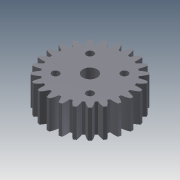
# Autodesk Inventor part: Spur Gear1
Saved by Autodesk Inventor 2015 (Build 190159000, 159)
## iProperties
Created: 2014-08-31
Part Number: Spur Gear1
Material: Steel
Document SubType Name: Modeling
Designer: shohei
Categories: <?xml version="1.0" encoding="UTF-16"?> <MemberInstance><Categories><FamilyTemplate><FamilyTemplateParameter ValueType="xs:double" Id="1" ObjectReferenceKey="da_z" ObjectType="kUserParameterObject"/><FamilyTemplateParameter ValueType="xs:double" Id="2" ObjectReferenceKey="da_b" ObjectType="kUserParameterObject"/><FamilyTemplateParameter ValueType="xs:double" Id="3" ObjectReferenceKey="da_beta" ObjectType="kUserParameterObject"/><FamilyTemplateParameter ValueType="xs:double" Id="4" ObjectReferenceKey="da_da" ObjectType="kUserParameterObject"/><FamilyTemplateParameter ValueType="xs:double" Id="5" ObjectReferenceKey="da_aw" ObjectType="kUserParameterObject"/><FamilyTemplateParameter ValueType="xs:string" Id="6" ObjectReferenceKey="EAIAABAAAACIAQAAAAAAAIAAAAAAAAAA" ObjectType="83910656" SubObjectId="SurfaceGeometry"/></FamilyTemplate><ParamToTemplateMap><ParamToTemplate CategoryParameter="//CategoryParameter[@InternalName='046C89C9-8512-4d59-83FE-43B91F4F132A']" TemplateParameter="1"/><ParamToTemplate CategoryParameter="//CategoryParameter[@InternalName='2552DF32-E462-4b46-AEBF-C6C7768E72AC']" TemplateParameter="2"/><ParamToTemplate CategoryParameter="//CategoryParameter[@InternalName='C9EE641D-15FC-4fae-A226-E94C4372FDD7']" TemplateParameter="3"/><ParamToTemplate><ParamToTemplate CategoryParameter="//CategoryParameter[@InternalName='00B6519A-459B-49c7-AD84-2E56D39A5744']" ConstantValue="0.000000"/></ParamToTemplate><ParamToTemplate><ParamToTemplate CategoryParameter="//CategoryParameter[@InternalName='04B31F0E-C7A6-4894-AA32-9629BEFACF47']" ConstantValue="1.000000"/></ParamToTemplate><ParamToTemplate><ParamToTemplate CategoryParameter="//CategoryParameter[@InternalName='43CBEC2E-7847-49e7-A936-2F7889FCB2D9']" ConstantValue="0.250000"/></ParamToTemplate><ParamToTemplate><ParamToTemplate CategoryParameter="//CategoryParameter[@InternalName='B1EFC894-105D-4ebd-86BF-FA20ED196853']" ConstantValue="0.350000"/></ParamToTemplate><ParamToTemplate><ParamToTemplate CategoryParameter="//CategoryParameter[@InternalName='51175063-3D10-4879-93E8-6246FE8B403D']" ConstantValue="2060000000.000000"/></ParamToTemplate><ParamToTemplate><ParamToTemplate CategoryParameter="//CategoryParameter[@InternalName='A3A52E27-4454-46a9-B0BD-C932399B70AF']" ConstantValue="0.300000"/></ParamToTemplate><ParamToTemplate><ParamToTemplate CategoryParameter="//CategoryParameter[@InternalName='91B76062-C214-41d9-B1B9-14D2AB99603D']" ConstantValue="0.225000"/></ParamToTemplate><ParamToTemplate><ParamToTemplate CategoryParameter="//CategoryParameter[@InternalName='374E806E-8B8A-4dda-A9AA-1039D6500AD2']" ConstantValue="4.444444"/></ParamToTemplate><ParamToTemplate><ParamToTemplate CategoryParameter="//CategoryParameter[@InternalName='2D373A89-B862-43d6-8D0B-0CBF12AB9F6C']" ConstantValue="0.349066"/></ParamToTemplate><ParamToTemplate CategoryParameter="//CategoryParameter[@InternalName='37777632-D6A2-4fac-9D53-DB8ACD95C989']" TemplateParameter="4"/><ParamToTemplate CategoryParameter="//CategoryParameter[@InternalName='FD1017F1-B727-4f7e-9707-0F86F1FF9423']" TemplateParameter="5"/><ParamToTemplate><ParamToTemplate CategoryParameter="//CategoryParameter[@InternalName='9E1B4470-B2D3-4ff1-B813-535BB4CDF51A']" ConstantValue="3520000.000000"/></ParamToTemplate><ParamToTemplate><ParamToTemplate CategoryParameter="//CategoryParameter[@InternalName='F8452263-BFF6-458c-9FB1-07C4B99E95CD']" ConstantValue="11400000.000000"/></ParamToTemplate><ParamToTemplate><ParamToTemplate CategoryParameter="//CategoryParameter[@InternalName='3E3BB259-FD49-497f-8171-6EBC954A3479']" ConstantValue="2.000000"/></ParamToTemplate><ParamToTemplate CategoryParameter="//CategoryParameter[@InternalName='27C3BAF2-7550-4e4b-AE2C-0DB134B7D9B7']" TemplateParameter="6"/></ParamToTemplateMap><Category DisplayName="Gear" InternalName="DC85795E-93AB-48d5-8EEE-5A27447B64BD" Mnemonic="Gear"><CategoryParameter DisplayName="z" InternalName="046C89C9-8512-4d59-83FE-43B91F4F132A" Mnemonic="z"/><CategoryParameter DisplayName="b" InternalName="2552DF32-E462-4b46-AEBF-C6C7768E72AC" Mnemonic="b"/><CategoryParameter DisplayName="||b|" InternalName="C9EE641D-15FC-4fae-A226-E94C4372FDD7" Mnemonic="beta"/><CategoryParameter DisplayName="x" InternalName="00B6519A-459B-49c7-AD84-2E56D39A5744" Mnemonic="x"/><CategoryParameter DisplayName="a*" InternalName="04B31F0E-C7A6-4894-AA32-9629BEFACF47" Mnemonic="a"/><CategoryParameter DisplayName="c*" InternalName="43CBEC2E-7847-49e7-A936-2F7889FCB2D9" Mnemonic="c"/><CategoryParameter DisplayName="r|.f|*" InternalName="B1EFC894-105D-4ebd-86BF-FA20ED196853" Mnemonic="rf"/><CategoryParameter DisplayName="E" InternalName="51175063-3D10-4879-93E8-6246FE8B403D" Mnemonic="E"/><CategoryParameter DisplayName="||m|" InternalName="A3A52E27-4454-46a9-B0BD-C932399B70AF" Mnemonic="mi"/><Category DisplayName="SpurGear" InternalName="26C5A22E-A91E-4dfd-A3B3-23CCAFAE1764" Mnemonic="SpurGear"><CategoryParameter DisplayName="m" InternalName="91B76062-C214-41d9-B1B9-14D2AB99603D" Mnemonic="m"/><CategoryParameter DisplayName="P" InternalName="374E806E-8B8A-4dda-A9AA-1039D6500AD2" Mnemonic="PP"/><CategoryParameter DisplayName="||a|" InternalName="2D373A89-B862-43d6-8D0B-0CBF12AB9F6C" Mnemonic="alpha"/><CategoryParameter DisplayName="d|.a|" InternalName="37777632-D6A2-4fac-9D53-DB8ACD95C989" Mnemonic="da"/><CategoryParameter DisplayName="a|.w|" InternalName="FD1017F1-B727-4f7e-9707-0F86F1FF9423" Mnemonic="aw"/><CategoryParameter DisplayName="||s||.Flim|" InternalName="9E1B4470-B2D3-4ff1-B813-535BB4CDF51A" Mnemonic="sFlim"/><CategoryParameter DisplayName="||s||.Hlim|" InternalName="F8452263-BFF6-458c-9FB1-07C4B99E95CD" Mnemonic="sHlim"/><CategoryParameter DisplayName="type" InternalName="3E3BB259-FD49-497f-8171-6EBC954A3479" Mnemonic="type"/><CategoryParameter DisplayName="PitchDiameter" InternalName="27C3BAF2-7550-4e4b-AE2C-0DB134B7D9B7" Mnemonic="IDS_PITCHDIAM"/></Category></Category></Categories></MemberInstance>
Density: 1 g/cm^3
Appearance: Steel
CustomPartVersion: 1
Author: shohei
Autodesk Inventor part; units mm, degrees
sketch "Block1" plane through (0, 0, 0) normal (0, 0, 1) x (1, 0, 0)
  arc A0 (1.1045, 29.446) -> (-1.1045, 29.446) centre (0, 0) ccw
  arc A1 (2.5646, 24.2724) -> (1.1045, 29.446) centre (-17.8247, 21.311) ccw
  arc A2 (3.805, 24.1091) -> (2.5646, 24.2724) centre (0, 0) ccw
  arc A3 (6.5543, 28.7285) -> (3.805, 24.1091) centre (22.733, 15.9715) ccw
  arc A4 (8.6881, 28.1567) -> (6.5543, 28.7285) centre (0, 0) ccw
  arc A5 (8.7594, 22.7816) -> (8.6881, 28.1567) centre (-11.7016, 25.1982) ccw
  arc A6 (9.9152, 22.3028) -> (8.7594, 22.7816) centre (0, 0) ccw
  arc A7 (13.7664, 26.0532) -> (9.9152, 22.3028) centre (26.0921, 9.5435) ccw
  arc A8 (15.6795, 24.9487) -> (13.7664, 26.0532) centre (0, 0) ccw
  arc A9 (14.3572, 19.7382) -> (15.6795, 24.9487) centre (-4.7811, 27.3682) ccw
  arc A10 (15.3497, 18.9766) -> (14.3572, 19.7382) centre (0, 0) ccw
  arc A11 (20.0404, 21.6024) -> (15.3497, 18.9766) centre (27.6731, 2.4652) ccw
  arc A12 (21.6024, 20.0404) -> (20.0404, 21.6024) centre (0, 0) ccw
  arc A13 (18.9766, 15.3497) -> (21.6024, 20.0404) centre (2.4652, 27.6731) ccw
  arc A14 (19.7382, 14.3572) -> (18.9766, 15.3497) centre (0, 0) ccw
  arc A15 (24.9487, 15.6795) -> (19.7382, 14.3572) centre (27.3682, -4.7811) ccw
  arc A16 (26.0532, 13.7664) -> (24.9487, 15.6795) centre (0, 0) ccw
  arc A17 (22.3028, 9.9152) -> (26.0532, 13.7664) centre (9.5435, 26.0921) ccw
  arc A18 (22.7816, 8.7594) -> (22.3028, 9.9152) centre (0, 0) ccw
  arc A19 (28.1567, 8.6881) -> (22.7816, 8.7594) centre (25.1982, -11.7016) ccw
  arc A20 (28.7285, 6.5543) -> (28.1567, 8.6881) centre (0, 0) ccw
  arc A21 (24.1091, 3.805) -> (28.7285, 6.5543) centre (15.9715, 22.733) ccw
  arc A22 (24.2724, 2.5646) -> (24.1091, 3.805) centre (0, 0) ccw
  arc A23 (29.446, 1.1045) -> (24.2724, 2.5646) centre (21.311, -17.8247) ccw
  arc A24 (29.446, -1.1045) -> (29.446, 1.1045) centre (0, 0) ccw
  arc A25 (24.2724, -2.5646) -> (29.446, -1.1045) centre (21.311, 17.8247) ccw
  arc A26 (24.1091, -3.805) -> (24.2724, -2.5646) centre (0, 0) ccw
  arc A27 (28.7285, -6.5543) -> (24.1091, -3.805) centre (15.9715, -22.733) ccw
  arc A28 (28.1567, -8.6881) -> (28.7285, -6.5543) centre (0, 0) ccw
  arc A29 (22.7816, -8.7594) -> (28.1567, -8.6881) centre (25.1982, 11.7016) ccw
  arc A30 (22.3028, -9.9152) -> (22.7816, -8.7594) centre (0, 0) ccw
  arc A31 (26.0532, -13.7664) -> (22.3028, -9.9152) centre (9.5435, -26.0921) ccw
  arc A32 (24.9487, -15.6795) -> (26.0532, -13.7664) centre (0, 0) ccw
  arc A33 (19.7382, -14.3572) -> (24.9487, -15.6795) centre (27.3682, 4.7811) ccw
  arc A34 (18.9766, -15.3497) -> (19.7382, -14.3572) centre (0, 0) ccw
  arc A35 (21.6024, -20.0404) -> (18.9766, -15.3497) centre (2.4652, -27.6731) ccw
  arc A36 (20.0404, -21.6024) -> (21.6024, -20.0404) centre (0, 0) ccw
  arc A37 (15.3497, -18.9766) -> (20.0404, -21.6024) centre (27.6731, -2.4652) ccw
  arc A38 (14.3572, -19.7382) -> (15.3497, -18.9766) centre (0, 0) ccw
  arc A39 (15.6795, -24.9487) -> (14.3572, -19.7382) centre (-4.7811, -27.3682) ccw
  arc A40 (13.7664, -26.0532) -> (15.6795, -24.9487) centre (0, 0) ccw
  arc A41 (9.9152, -22.3028) -> (13.7664, -26.0532) centre (26.0921, -9.5435) ccw
  arc A42 (8.7594, -22.7816) -> (9.9152, -22.3028) centre (0, 0) ccw
  arc A43 (8.6881, -28.1567) -> (8.7594, -22.7816) centre (-11.7016, -25.1982) ccw
  arc A44 (6.5543, -28.7285) -> (8.6881, -28.1567) centre (0, 0) ccw
  arc A45 (3.805, -24.1091) -> (6.5543, -28.7285) centre (22.733, -15.9715) ccw
  arc A46 (2.5646, -24.2724) -> (3.805, -24.1091) centre (0, 0) ccw
  arc A47 (1.1045, -29.446) -> (2.5646, -24.2724) centre (-17.8247, -21.311) ccw
  arc A48 (-1.1045, -29.446) -> (1.1045, -29.446) centre (0, 0) ccw
  arc A49 (-2.5646, -24.2724) -> (-1.1045, -29.446) centre (17.8247, -21.311) ccw
  arc A50 (-3.805, -24.1091) -> (-2.5646, -24.2724) centre (0, 0) ccw
  arc A51 (-6.5543, -28.7285) -> (-3.805, -24.1091) centre (-22.733, -15.9715) ccw
  arc A52 (-8.6881, -28.1567) -> (-6.5543, -28.7285) centre (0, 0) ccw
  arc A53 (-8.7594, -22.7816) -> (-8.6881, -28.1567) centre (11.7016, -25.1982) ccw
  arc A54 (-9.9152, -22.3028) -> (-8.7594, -22.7816) centre (0, 0) ccw
  arc A55 (-13.7664, -26.0532) -> (-9.9152, -22.3028) centre (-26.0921, -9.5435) ccw
  arc A56 (-15.6795, -24.9487) -> (-13.7664, -26.0532) centre (0, 0) ccw
  arc A57 (-14.3572, -19.7382) -> (-15.6795, -24.9487) centre (4.7811, -27.3682) ccw
  arc A58 (-15.3497, -18.9766) -> (-14.3572, -19.7382) centre (0, 0) ccw
  arc A59 (-20.0404, -21.6024) -> (-15.3497, -18.9766) centre (-27.6731, -2.4652) ccw
  arc A60 (-21.6024, -20.0404) -> (-20.0404, -21.6024) centre (0, 0) ccw
  arc A61 (-18.9766, -15.3497) -> (-21.6024, -20.0404) centre (-2.4652, -27.6731) ccw
  arc A62 (-19.7382, -14.3572) -> (-18.9766, -15.3497) centre (0, 0) ccw
  arc A63 (-24.9487, -15.6795) -> (-19.7382, -14.3572) centre (-27.3682, 4.7811) ccw
  arc A64 (-26.0532, -13.7664) -> (-24.9487, -15.6795) centre (0, 0) ccw
  arc A65 (-22.3028, -9.9152) -> (-26.0532, -13.7664) centre (-9.5435, -26.0921) ccw
  arc A66 (-22.7816, -8.7594) -> (-22.3028, -9.9152) centre (0, 0) ccw
  arc A67 (-28.1567, -8.6881) -> (-22.7816, -8.7594) centre (-25.1982, 11.7016) ccw
  arc A68 (-28.7285, -6.5543) -> (-28.1567, -8.6881) centre (0, 0) ccw
  arc A69 (-24.1091, -3.805) -> (-28.7285, -6.5543) centre (-15.9715, -22.733) ccw
  arc A70 (-24.2724, -2.5646) -> (-24.1091, -3.805) centre (0, 0) ccw
  arc A71 (-29.446, -1.1045) -> (-24.2724, -2.5646) centre (-21.311, 17.8247) ccw
  arc A72 (-29.446, 1.1045) -> (-29.446, -1.1045) centre (0, 0) ccw
  arc A73 (-24.2724, 2.5646) -> (-29.446, 1.1045) centre (-21.311, -17.8247) ccw
  arc A74 (-24.1091, 3.805) -> (-24.2724, 2.5646) centre (0, 0) ccw
  arc A75 (-28.7285, 6.5543) -> (-24.1091, 3.805) centre (-15.9715, 22.733) ccw
  arc A76 (-28.1567, 8.6881) -> (-28.7285, 6.5543) centre (0, 0) ccw
  arc A77 (-22.7816, 8.7594) -> (-28.1567, 8.6881) centre (-25.1982, -11.7016) ccw
  arc A78 (-22.3028, 9.9152) -> (-22.7816, 8.7594) centre (0, 0) ccw
  arc A79 (-26.0532, 13.7664) -> (-22.3028, 9.9152) centre (-9.5435, 26.0921) ccw
  arc A80 (-24.9487, 15.6795) -> (-26.0532, 13.7664) centre (0, 0) ccw
  arc A81 (-19.7382, 14.3572) -> (-24.9487, 15.6795) centre (-27.3682, -4.7811) ccw
  arc A82 (-18.9766, 15.3497) -> (-19.7382, 14.3572) centre (0, 0) ccw
  arc A83 (-21.6024, 20.0404) -> (-18.9766, 15.3497) centre (-2.4652, 27.6731) ccw
  arc A84 (-20.0404, 21.6024) -> (-21.6024, 20.0404) centre (0, 0) ccw
  arc A85 (-15.3497, 18.9766) -> (-20.0404, 21.6024) centre (-27.6731, 2.4652) ccw
  arc A86 (-14.3572, 19.7382) -> (-15.3497, 18.9766) centre (0, 0) ccw
  arc A87 (-15.6795, 24.9487) -> (-14.3572, 19.7382) centre (4.7811, 27.3682) ccw
  arc A88 (-13.7664, 26.0532) -> (-15.6795, 24.9487) centre (0, 0) ccw
  arc A89 (-9.9152, 22.3028) -> (-13.7664, 26.0532) centre (-26.0921, 9.5435) ccw
  arc A90 (-8.7594, 22.7816) -> (-9.9152, 22.3028) centre (0, 0) ccw
  arc A91 (-8.6881, 28.1567) -> (-8.7594, 22.7816) centre (11.7016, 25.1982) ccw
  arc A92 (-6.5543, 28.7285) -> (-8.6881, 28.1567) centre (0, 0) ccw
  arc A93 (-3.805, 24.1091) -> (-6.5543, 28.7285) centre (-22.733, 15.9715) ccw
  arc A94 (-2.5646, 24.2724) -> (-3.805, 24.1091) centre (0, 0) ccw
  arc A95 (-1.1045, 29.446) -> (-2.5646, 24.2724) centre (17.8247, 21.311) ccw
  circle A96 centre (0, 0) radius 5.22
  circle A97 centre (-12, 12) radius 2.72
  circle A98 centre (-12, -12) radius 2.72
  circle A99 centre (12, 12) radius 2.72
  circle A100 centre (12, -12) radius 2.72
  point P0 (0, 0)
sketch "Sketch1" plane through (0, 0, 0) normal (0, 0, 1) x (1, 0, 0)
  circle A0 centre (0, 0) radius 29.2467
  dimension "d0" = 58.4933
  constraints: 1 centre point
  measures "d0" diameter of A0
extrude "Extrusion1" add sketch "Sketch1" along normal blind 20
ref_plane "Work Plane2" through (0, 0, 10) normal (0, 0, 1) x (1, 0, 0)
sketch "Sketch2" plane through (0, 0, 0) normal (0, 0, -1) x (-1, 0, 0)
  circle A0 centre (0, 0) radius 29.2467 projected
  circle A1 centre (0, 0) radius 27.0968
  dimension "d3" = 54.1936
  constraints: 1 centre point, 1 coincident
  measures "d3" diameter of A1
surface extrude "Pitch Diameter" sketch "Sketch2" against normal through all shown no curves A1
ref_plane "Work Plane8" through (0, 0, 0) normal (0.9914449, 0.1305262, 0) x (0, 0, 1)
ref_plane "Work Plane9" through (0, 0, 0) normal (1, 0, 0) x (0, 1, 0)
spur gear teeth "Spur Gear" teeth 24 pitch diameter 54 tip diameter 58.4933 root diameter 48.375 face width 20 start plane through (0, 0, 0) normal (0, 0, -1) x (-1, 0, 0)
sketch "Sketch3" plane through (0, 0, 0) normal (0, 0, -1) x (-1, 0, 0)
  circle A0 centre (0, 0) radius 5
  line L0 (40.9453, 0) -> (-40.9453, 0) projected
  line L1 (0, -40.9453) -> (0, 40.9453) projected
  circle A1 centre (12, 12) radius 2.5
  circle A2 centre (-12, 12) radius 2.5
  circle A3 centre (12, -12) radius 2.5
  circle A4 centre (-12, -12) radius 2.5
  dimension "d49" = 10
  dimension "d52" = 5
  dimension "d53" = 12
  dimension "d54" = 12
  constraints: 5 centre point, 3 symmetric about line, 1 coincident, 3 other
  measures "d49" diameter of A0
  measures "d52" diameter of A1
  measures "d53" distance from line of L1 A1.centre
  measures "d54" distance from line of L0 A1.centre
extrude "Extrusion3" cut sketch "Sketch3" against normal through all
sketch "Sketch4" plane through (0, 0, 20) normal (0, 0, 1) x (1, 0, 0)
  circle A0 centre (12, -12) radius 2.5 projected
  circle A1 centre (12, 12) radius 2.5 projected
  circle A2 centre (-12, 12) radius 2.5 projected
  circle A3 centre (-12, -12) radius 2.5 projected
  circle A4 centre (0, 0) radius 5 projected
  arc A5 (-8.4899, 27.9873) -> (-8.52, 22.6372) centre (11.7016, 25.1982) ccw projected
  arc A6 (-8.52, 22.6372) -> (-9.9824, 22.0315) centre (0, 0) ccw projected
  arc A7 (-9.9824, 22.0315) -> (-13.7868, 25.7933) centre (-26.0921, 9.5435) ccw projected
  arc A8 (-13.7868, 25.7933) -> (-15.4442, 24.8363) centre (0, 0) ccw projected
  arc A9 (-15.4442, 24.8363) -> (-14.0887, 19.6607) centre (4.7811, 27.3682) ccw projected
  arc A10 (-14.0887, 19.6607) -> (-15.3444, 18.6972) centre (0, 0) ccw projected
  arc A11 (-15.3444, 18.6972) -> (-19.9928, 21.3461) centre (-27.6731, 2.4652) ccw projected
  arc A12 (-19.9928, 21.3461) -> (-21.3461, 19.9928) centre (0, 0) ccw projected
  arc A13 (-21.3461, 19.9928) -> (-18.6972, 15.3444) centre (-2.4652, 27.6731) ccw projected
  arc A14 (-18.6972, 15.3444) -> (-19.6607, 14.0887) centre (0, 0) ccw projected
  arc A15 (-19.6607, 14.0887) -> (-24.8363, 15.4442) centre (-27.3682, -4.7811) ccw projected
  arc A16 (-24.8363, 15.4442) -> (-25.7933, 13.7868) centre (0, 0) ccw projected
  arc A17 (-25.7933, 13.7868) -> (-22.0315, 9.9824) centre (-9.5435, 26.0921) ccw projected
  arc A18 (-22.0315, 9.9824) -> (-22.6372, 8.52) centre (0, 0) ccw projected
  arc A19 (-22.6372, 8.52) -> (-27.9873, 8.4899) centre (-25.1982, -11.7016) ccw projected
  arc A20 (-27.9873, 8.4899) -> (-28.4826, 6.6412) centre (0, 0) ccw projected
  arc A21 (-28.4826, 6.6412) -> (-23.8644, 3.94) centre (-15.9715, 22.733) ccw projected
  arc A22 (-23.8644, 3.94) -> (-24.071, 2.3708) centre (0, 0) ccw projected
  arc A23 (-24.071, 2.3708) -> (-29.231, 0.9569) centre (-21.311, -17.8247) ccw projected
  arc A24 (-29.231, 0.9569) -> (-29.231, -0.9569) centre (0, 0) ccw projected
  arc A25 (-29.231, -0.9569) -> (-24.071, -2.3708) centre (-21.311, 17.8247) ccw projected
  arc A26 (-24.071, -2.3708) -> (-23.8644, -3.94) centre (0, 0) ccw projected
  arc A27 (-23.8644, -3.94) -> (-28.4826, -6.6412) centre (-15.9715, -22.733) ccw projected
  arc A28 (-28.4826, -6.6412) -> (-27.9873, -8.4899) centre (0, 0) ccw projected
  arc A29 (-27.9873, -8.4899) -> (-22.6372, -8.52) centre (-25.1982, 11.7016) ccw projected
  arc A30 (-22.6372, -8.52) -> (-22.0315, -9.9824) centre (0, 0) ccw projected
  arc A31 (-22.0315, -9.9824) -> (-25.7933, -13.7868) centre (-9.5435, -26.0921) ccw projected
  arc A32 (-25.7933, -13.7868) -> (-24.8363, -15.4442) centre (0, 0) ccw projected
  arc A33 (-24.8363, -15.4442) -> (-19.6607, -14.0887) centre (-27.3682, 4.7811) ccw projected
  arc A34 (-19.6607, -14.0887) -> (-18.6972, -15.3444) centre (0, 0) ccw projected
  arc A35 (-18.6972, -15.3444) -> (-21.3461, -19.9928) centre (-2.4652, -27.6731) ccw projected
  arc A36 (-21.3461, -19.9928) -> (-19.9928, -21.3461) centre (0, 0) ccw projected
  arc A37 (-19.9928, -21.3461) -> (-15.3444, -18.6972) centre (-27.6731, -2.4652) ccw projected
  arc A38 (-15.3444, -18.6972) -> (-14.0887, -19.6607) centre (0, 0) ccw projected
  arc A39 (-14.0887, -19.6607) -> (-15.4442, -24.8363) centre (4.7811, -27.3682) ccw projected
  arc A40 (-15.4442, -24.8363) -> (-13.7868, -25.7933) centre (0, 0) ccw projected
  arc A41 (-13.7868, -25.7933) -> (-9.9824, -22.0315) centre (-26.0921, -9.5435) ccw projected
  arc A42 (-9.9824, -22.0315) -> (-8.52, -22.6372) centre (0, 0) ccw projected
  arc A43 (-8.52, -22.6372) -> (-8.4899, -27.9873) centre (11.7016, -25.1982) ccw projected
  arc A44 (-8.4899, -27.9873) -> (-6.6412, -28.4826) centre (0, 0) ccw projected
  arc A45 (-6.6412, -28.4826) -> (-3.94, -23.8644) centre (-22.733, -15.9715) ccw projected
  arc A46 (-3.94, -23.8644) -> (-2.3708, -24.071) centre (0, 0) ccw projected
  arc A47 (-2.3708, -24.071) -> (-0.9569, -29.231) centre (17.8247, -21.311) ccw projected
  arc A48 (-0.9569, -29.231) -> (0.9569, -29.231) centre (0, 0) ccw projected
  arc A49 (0.9569, -29.231) -> (2.3708, -24.071) centre (-17.8247, -21.311) ccw projected
  arc A50 (2.3708, -24.071) -> (3.94, -23.8644) centre (0, 0) ccw projected
  arc A51 (3.94, -23.8644) -> (6.6412, -28.4826) centre (22.733, -15.9715) ccw projected
  arc A52 (6.6412, -28.4826) -> (8.4899, -27.9873) centre (0, 0) ccw projected
  arc A53 (8.4899, -27.9873) -> (8.52, -22.6372) centre (-11.7016, -25.1982) ccw projected
  arc A54 (8.52, -22.6372) -> (9.9824, -22.0315) centre (0, 0) ccw projected
  arc A55 (9.9824, -22.0315) -> (13.7868, -25.7933) centre (26.0921, -9.5435) ccw projected
  arc A56 (13.7868, -25.7933) -> (15.4442, -24.8363) centre (0, 0) ccw projected
  arc A57 (15.4442, -24.8363) -> (14.0887, -19.6607) centre (-4.7811, -27.3682) ccw projected
  arc A58 (14.0887, -19.6607) -> (15.3444, -18.6972) centre (0, 0) ccw projected
  arc A59 (15.3444, -18.6972) -> (19.9928, -21.3461) centre (27.6731, -2.4652) ccw projected
  arc A60 (19.9928, -21.3461) -> (21.3461, -19.9928) centre (0, 0) ccw projected
  arc A61 (21.3461, -19.9928) -> (18.6972, -15.3444) centre (2.4652, -27.6731) ccw projected
  arc A62 (18.6972, -15.3444) -> (19.6607, -14.0887) centre (0, 0) ccw projected
  arc A63 (19.6607, -14.0887) -> (24.8363, -15.4442) centre (27.3682, 4.7811) ccw projected
  arc A64 (24.8363, -15.4442) -> (25.7933, -13.7868) centre (0, 0) ccw projected
  arc A65 (25.7933, -13.7868) -> (22.0315, -9.9824) centre (9.5435, -26.0921) ccw projected
  arc A66 (22.0315, -9.9824) -> (22.6372, -8.52) centre (0, 0) ccw projected
  arc A67 (22.6372, -8.52) -> (27.9873, -8.4899) centre (25.1982, 11.7016) ccw projected
  arc A68 (27.9873, -8.4899) -> (28.4826, -6.6412) centre (0, 0) ccw projected
  arc A69 (28.4826, -6.6412) -> (23.8644, -3.94) centre (15.9715, -22.733) ccw projected
  arc A70 (23.8644, -3.94) -> (24.071, -2.3708) centre (0, 0) ccw projected
  arc A71 (24.071, -2.3708) -> (29.231, -0.9569) centre (21.311, 17.8247) ccw projected
  arc A72 (29.231, -0.9569) -> (29.231, 0.9569) centre (0, 0) ccw projected
  arc A73 (29.231, 0.9569) -> (24.071, 2.3708) centre (21.311, -17.8247) ccw projected
  arc A74 (24.071, 2.3708) -> (23.8644, 3.94) centre (0, 0) ccw projected
  arc A75 (23.8644, 3.94) -> (28.4826, 6.6412) centre (15.9715, 22.733) ccw projected
  arc A76 (28.4826, 6.6412) -> (27.9873, 8.4899) centre (0, 0) ccw projected
  arc A77 (27.9873, 8.4899) -> (22.6372, 8.52) centre (25.1982, -11.7016) ccw projected
  arc A78 (22.6372, 8.52) -> (22.0315, 9.9824) centre (0, 0) ccw projected
  arc A79 (22.0315, 9.9824) -> (25.7933, 13.7868) centre (9.5435, 26.0921) ccw projected
  arc A80 (25.7933, 13.7868) -> (24.8363, 15.4442) centre (0, 0) ccw projected
  arc A81 (24.8363, 15.4442) -> (19.6607, 14.0887) centre (27.3682, -4.7811) ccw projected
  arc A82 (19.6607, 14.0887) -> (18.6972, 15.3444) centre (0, 0) ccw projected
  arc A83 (18.6972, 15.3444) -> (21.3461, 19.9928) centre (2.4652, 27.6731) ccw projected
  arc A84 (21.3461, 19.9928) -> (19.9928, 21.3461) centre (0, 0) ccw projected
  arc A85 (19.9928, 21.3461) -> (15.3444, 18.6972) centre (27.6731, 2.4652) ccw projected
  arc A86 (15.3444, 18.6972) -> (14.0887, 19.6607) centre (0, 0) ccw projected
  arc A87 (14.0887, 19.6607) -> (15.4442, 24.8363) centre (-4.7811, 27.3682) ccw projected
  arc A88 (15.4442, 24.8363) -> (13.7868, 25.7933) centre (0, 0) ccw projected
  arc A89 (13.7868, 25.7933) -> (9.9824, 22.0315) centre (26.0921, 9.5435) ccw projected
  arc A90 (9.9824, 22.0315) -> (8.52, 22.6372) centre (0, 0) ccw projected
  arc A91 (8.52, 22.6372) -> (8.4899, 27.9873) centre (-11.7016, 25.1982) ccw projected
  arc A92 (8.4899, 27.9873) -> (6.6412, 28.4826) centre (0, 0) ccw projected
  arc A93 (6.6412, 28.4826) -> (3.94, 23.8644) centre (22.733, 15.9715) ccw projected
  arc A94 (3.94, 23.8644) -> (2.3708, 24.071) centre (0, 0) ccw projected
  arc A95 (2.3708, 24.071) -> (0.9569, 29.231) centre (-17.8247, 21.311) ccw projected
  arc A96 (0.9569, 29.231) -> (-0.9569, 29.231) centre (0, 0) ccw projected
  arc A97 (-0.9569, 29.231) -> (-2.3708, 24.071) centre (17.8247, 21.311) ccw projected
  arc A98 (-2.3708, 24.071) -> (-3.94, 23.8644) centre (0, 0) ccw projected
  arc A99 (-3.94, 23.8644) -> (-6.6412, 28.4826) centre (-22.733, 15.9715) ccw projected
  arc A100 (-6.6412, 28.4826) -> (-8.4899, 27.9873) centre (0, 0) ccw projected
  arc A101 (1.1045, 29.446) -> (-1.1045, 29.446) centre (0, 0) ccw
  arc A102 (2.5646, 24.2724) -> (1.1045, 29.446) centre (-17.8247, 21.311) ccw
  arc A103 (3.805, 24.1091) -> (2.5646, 24.2724) centre (0, 0) ccw
  arc A104 (6.5543, 28.7285) -> (3.805, 24.1091) centre (22.733, 15.9715) ccw
  arc A105 (8.6881, 28.1567) -> (6.5543, 28.7285) centre (0, 0) ccw
  arc A106 (8.7594, 22.7816) -> (8.6881, 28.1567) centre (-11.7016, 25.1982) ccw
  arc A107 (9.9152, 22.3028) -> (8.7594, 22.7816) centre (0, 0) ccw
  arc A108 (13.7664, 26.0532) -> (9.9152, 22.3028) centre (26.0921, 9.5435) ccw
  arc A109 (15.6795, 24.9487) -> (13.7664, 26.0532) centre (0, 0) ccw
  arc A110 (14.3572, 19.7382) -> (15.6795, 24.9487) centre (-4.7811, 27.3682) ccw
  arc A111 (15.3497, 18.9766) -> (14.3572, 19.7382) centre (0, 0) ccw
  arc A112 (20.0404, 21.6024) -> (15.3497, 18.9766) centre (27.6731, 2.4652) ccw
  arc A113 (21.6024, 20.0404) -> (20.0404, 21.6024) centre (0, 0) ccw
  arc A114 (18.9766, 15.3497) -> (21.6024, 20.0404) centre (2.4652, 27.6731) ccw
  arc A115 (19.7382, 14.3572) -> (18.9766, 15.3497) centre (0, 0) ccw
  arc A116 (24.9487, 15.6795) -> (19.7382, 14.3572) centre (27.3682, -4.7811) ccw
  arc A117 (26.0532, 13.7664) -> (24.9487, 15.6795) centre (0, 0) ccw
  arc A118 (22.3028, 9.9152) -> (26.0532, 13.7664) centre (9.5435, 26.0921) ccw
  arc A119 (22.7816, 8.7594) -> (22.3028, 9.9152) centre (0, 0) ccw
  arc A120 (28.1567, 8.6881) -> (22.7816, 8.7594) centre (25.1982, -11.7016) ccw
  arc A121 (28.7285, 6.5543) -> (28.1567, 8.6881) centre (0, 0) ccw
  arc A122 (24.1091, 3.805) -> (28.7285, 6.5543) centre (15.9715, 22.733) ccw
  arc A123 (24.2724, 2.5646) -> (24.1091, 3.805) centre (0, 0) ccw
  arc A124 (29.446, 1.1045) -> (24.2724, 2.5646) centre (21.311, -17.8247) ccw
  arc A125 (29.446, -1.1045) -> (29.446, 1.1045) centre (0, 0) ccw
  arc A126 (24.2724, -2.5646) -> (29.446, -1.1045) centre (21.311, 17.8247) ccw
  arc A127 (24.1091, -3.805) -> (24.2724, -2.5646) centre (0, 0) ccw
  arc A128 (28.7285, -6.5543) -> (24.1091, -3.805) centre (15.9715, -22.733) ccw
  arc A129 (28.1567, -8.6881) -> (28.7285, -6.5543) centre (0, 0) ccw
  arc A130 (22.7816, -8.7594) -> (28.1567, -8.6881) centre (25.1982, 11.7016) ccw
  arc A131 (22.3028, -9.9152) -> (22.7816, -8.7594) centre (0, 0) ccw
  arc A132 (26.0532, -13.7664) -> (22.3028, -9.9152) centre (9.5435, -26.0921) ccw
  arc A133 (24.9487, -15.6795) -> (26.0532, -13.7664) centre (0, 0) ccw
  arc A134 (19.7382, -14.3572) -> (24.9487, -15.6795) centre (27.3682, 4.7811) ccw
  arc A135 (18.9766, -15.3497) -> (19.7382, -14.3572) centre (0, 0) ccw
  arc A136 (21.6024, -20.0404) -> (18.9766, -15.3497) centre (2.4652, -27.6731) ccw
  arc A137 (20.0404, -21.6024) -> (21.6024, -20.0404) centre (0, 0) ccw
  arc A138 (15.3497, -18.9766) -> (20.0404, -21.6024) centre (27.6731, -2.4652) ccw
  arc A139 (14.3572, -19.7382) -> (15.3497, -18.9766) centre (0, 0) ccw
  arc A140 (15.6795, -24.9487) -> (14.3572, -19.7382) centre (-4.7811, -27.3682) ccw
  arc A141 (13.7664, -26.0532) -> (15.6795, -24.9487) centre (0, 0) ccw
  arc A142 (9.9152, -22.3028) -> (13.7664, -26.0532) centre (26.0921, -9.5435) ccw
  arc A143 (8.7594, -22.7816) -> (9.9152, -22.3028) centre (0, 0) ccw
  arc A144 (8.6881, -28.1567) -> (8.7594, -22.7816) centre (-11.7016, -25.1982) ccw
  arc A145 (6.5543, -28.7285) -> (8.6881, -28.1567) centre (0, 0) ccw
  arc A146 (3.805, -24.1091) -> (6.5543, -28.7285) centre (22.733, -15.9715) ccw
  arc A147 (2.5646, -24.2724) -> (3.805, -24.1091) centre (0, 0) ccw
  arc A148 (1.1045, -29.446) -> (2.5646, -24.2724) centre (-17.8247, -21.311) ccw
  arc A149 (-1.1045, -29.446) -> (1.1045, -29.446) centre (0, 0) ccw
  arc A150 (-2.5646, -24.2724) -> (-1.1045, -29.446) centre (17.8247, -21.311) ccw
  arc A151 (-3.805, -24.1091) -> (-2.5646, -24.2724) centre (0, 0) ccw
  arc A152 (-6.5543, -28.7285) -> (-3.805, -24.1091) centre (-22.733, -15.9715) ccw
  arc A153 (-8.6881, -28.1567) -> (-6.5543, -28.7285) centre (0, 0) ccw
  arc A154 (-8.7594, -22.7816) -> (-8.6881, -28.1567) centre (11.7016, -25.1982) ccw
  arc A155 (-9.9152, -22.3028) -> (-8.7594, -22.7816) centre (0, 0) ccw
  arc A156 (-13.7664, -26.0532) -> (-9.9152, -22.3028) centre (-26.0921, -9.5435) ccw
  arc A157 (-15.6795, -24.9487) -> (-13.7664, -26.0532) centre (0, 0) ccw
  arc A158 (-14.3572, -19.7382) -> (-15.6795, -24.9487) centre (4.7811, -27.3682) ccw
  arc A159 (-15.3497, -18.9766) -> (-14.3572, -19.7382) centre (0, 0) ccw
  arc A160 (-20.0404, -21.6024) -> (-15.3497, -18.9766) centre (-27.6731, -2.4652) ccw
  arc A161 (-21.6024, -20.0404) -> (-20.0404, -21.6024) centre (0, 0) ccw
  arc A162 (-18.9766, -15.3497) -> (-21.6024, -20.0404) centre (-2.4652, -27.6731) ccw
  arc A163 (-19.7382, -14.3572) -> (-18.9766, -15.3497) centre (0, 0) ccw
  arc A164 (-24.9487, -15.6795) -> (-19.7382, -14.3572) centre (-27.3682, 4.7811) ccw
  arc A165 (-26.0532, -13.7664) -> (-24.9487, -15.6795) centre (0, 0) ccw
  arc A166 (-22.3028, -9.9152) -> (-26.0532, -13.7664) centre (-9.5435, -26.0921) ccw
  arc A167 (-22.7816, -8.7594) -> (-22.3028, -9.9152) centre (0, 0) ccw
  arc A168 (-28.1567, -8.6881) -> (-22.7816, -8.7594) centre (-25.1982, 11.7016) ccw
  arc A169 (-28.7285, -6.5543) -> (-28.1567, -8.6881) centre (0, 0) ccw
  arc A170 (-24.1091, -3.805) -> (-28.7285, -6.5543) centre (-15.9715, -22.733) ccw
  arc A171 (-24.2724, -2.5646) -> (-24.1091, -3.805) centre (0, 0) ccw
  arc A172 (-29.446, -1.1045) -> (-24.2724, -2.5646) centre (-21.311, 17.8247) ccw
  arc A173 (-29.446, 1.1045) -> (-29.446, -1.1045) centre (0, 0) ccw
  arc A174 (-24.2724, 2.5646) -> (-29.446, 1.1045) centre (-21.311, -17.8247) ccw
  arc A175 (-24.1091, 3.805) -> (-24.2724, 2.5646) centre (0, 0) ccw
  arc A176 (-28.7285, 6.5543) -> (-24.1091, 3.805) centre (-15.9715, 22.733) ccw
  arc A177 (-28.1567, 8.6881) -> (-28.7285, 6.5543) centre (0, 0) ccw
  arc A178 (-22.7816, 8.7594) -> (-28.1567, 8.6881) centre (-25.1982, -11.7016) ccw
  arc A179 (-22.3028, 9.9152) -> (-22.7816, 8.7594) centre (0, 0) ccw
  arc A180 (-26.0532, 13.7664) -> (-22.3028, 9.9152) centre (-9.5435, 26.0921) ccw
  arc A181 (-24.9487, 15.6795) -> (-26.0532, 13.7664) centre (0, 0) ccw
  arc A182 (-19.7382, 14.3572) -> (-24.9487, 15.6795) centre (-27.3682, -4.7811) ccw
  arc A183 (-18.9766, 15.3497) -> (-19.7382, 14.3572) centre (0, 0) ccw
  arc A184 (-21.6024, 20.0404) -> (-18.9766, 15.3497) centre (-2.4652, 27.6731) ccw
  arc A185 (-20.0404, 21.6024) -> (-21.6024, 20.0404) centre (0, 0) ccw
  arc A186 (-15.3497, 18.9766) -> (-20.0404, 21.6024) centre (-27.6731, 2.4652) ccw
  arc A187 (-14.3572, 19.7382) -> (-15.3497, 18.9766) centre (0, 0) ccw
  arc A188 (-15.6795, 24.9487) -> (-14.3572, 19.7382) centre (4.7811, 27.3682) ccw
  arc A189 (-13.7664, 26.0532) -> (-15.6795, 24.9487) centre (0, 0) ccw
  arc A190 (-9.9152, 22.3028) -> (-13.7664, 26.0532) centre (-26.0921, 9.5435) ccw
  arc A191 (-8.7594, 22.7816) -> (-9.9152, 22.3028) centre (0, 0) ccw
  arc A192 (-8.6881, 28.1567) -> (-8.7594, 22.7816) centre (11.7016, 25.1982) ccw
  arc A193 (-6.5543, 28.7285) -> (-8.6881, 28.1567) centre (0, 0) ccw
  arc A194 (-3.805, 24.1091) -> (-6.5543, 28.7285) centre (-22.733, 15.9715) ccw
  arc A195 (-2.5646, 24.2724) -> (-3.805, 24.1091) centre (0, 0) ccw
  arc A196 (-1.1045, 29.446) -> (-2.5646, 24.2724) centre (17.8247, 21.311) ccw
  circle A197 centre (0, 0) radius 5.22
  circle A198 centre (-12, 12) radius 2.72
  circle A199 centre (-12, -12) radius 2.72
  circle A200 centre (12, 12) radius 2.72
  circle A201 centre (12, -12) radius 2.72
  constraints: 196 other
sketch "DXF" plane through (0, 0, 0) normal (0, 0, 1) x (1, 0, 0)
  arc A0 (1.1045, 29.446) -> (-1.1045, 29.446) centre (0, 0) ccw
  arc A1 (2.5646, 24.2724) -> (1.1045, 29.446) centre (-17.8247, 21.311) ccw
  arc A2 (3.805, 24.1091) -> (2.5646, 24.2724) centre (0, 0) ccw
  arc A3 (6.5543, 28.7285) -> (3.805, 24.1091) centre (22.733, 15.9715) ccw
  arc A4 (8.6881, 28.1567) -> (6.5543, 28.7285) centre (0, 0) ccw
  arc A5 (8.7594, 22.7816) -> (8.6881, 28.1567) centre (-11.7016, 25.1982) ccw
  arc A6 (9.9152, 22.3028) -> (8.7594, 22.7816) centre (0, 0) ccw
  arc A7 (13.7664, 26.0532) -> (9.9152, 22.3028) centre (26.0921, 9.5435) ccw
  arc A8 (15.6795, 24.9487) -> (13.7664, 26.0532) centre (0, 0) ccw
  arc A9 (14.3572, 19.7382) -> (15.6795, 24.9487) centre (-4.7811, 27.3682) ccw
  arc A10 (15.3497, 18.9766) -> (14.3572, 19.7382) centre (0, 0) ccw
  arc A11 (20.0404, 21.6024) -> (15.3497, 18.9766) centre (27.6731, 2.4652) ccw
  arc A12 (21.6024, 20.0404) -> (20.0404, 21.6024) centre (0, 0) ccw
  arc A13 (18.9766, 15.3497) -> (21.6024, 20.0404) centre (2.4652, 27.6731) ccw
  arc A14 (19.7382, 14.3572) -> (18.9766, 15.3497) centre (0, 0) ccw
  arc A15 (24.9487, 15.6795) -> (19.7382, 14.3572) centre (27.3682, -4.7811) ccw
  arc A16 (26.0532, 13.7664) -> (24.9487, 15.6795) centre (0, 0) ccw
  arc A17 (22.3028, 9.9152) -> (26.0532, 13.7664) centre (9.5435, 26.0921) ccw
  arc A18 (22.7816, 8.7594) -> (22.3028, 9.9152) centre (0, 0) ccw
  arc A19 (28.1567, 8.6881) -> (22.7816, 8.7594) centre (25.1982, -11.7016) ccw
  arc A20 (28.7285, 6.5543) -> (28.1567, 8.6881) centre (0, 0) ccw
  arc A21 (24.1091, 3.805) -> (28.7285, 6.5543) centre (15.9715, 22.733) ccw
  arc A22 (24.2724, 2.5646) -> (24.1091, 3.805) centre (0, 0) ccw
  arc A23 (29.446, 1.1045) -> (24.2724, 2.5646) centre (21.311, -17.8247) ccw
  arc A24 (29.446, -1.1045) -> (29.446, 1.1045) centre (0, 0) ccw
  arc A25 (24.2724, -2.5646) -> (29.446, -1.1045) centre (21.311, 17.8247) ccw
  arc A26 (24.1091, -3.805) -> (24.2724, -2.5646) centre (0, 0) ccw
  arc A27 (28.7285, -6.5543) -> (24.1091, -3.805) centre (15.9715, -22.733) ccw
  arc A28 (28.1567, -8.6881) -> (28.7285, -6.5543) centre (0, 0) ccw
  arc A29 (22.7816, -8.7594) -> (28.1567, -8.6881) centre (25.1982, 11.7016) ccw
  arc A30 (22.3028, -9.9152) -> (22.7816, -8.7594) centre (0, 0) ccw
  arc A31 (26.0532, -13.7664) -> (22.3028, -9.9152) centre (9.5435, -26.0921) ccw
  arc A32 (24.9487, -15.6795) -> (26.0532, -13.7664) centre (0, 0) ccw
  arc A33 (19.7382, -14.3572) -> (24.9487, -15.6795) centre (27.3682, 4.7811) ccw
  arc A34 (18.9766, -15.3497) -> (19.7382, -14.3572) centre (0, 0) ccw
  arc A35 (21.6024, -20.0404) -> (18.9766, -15.3497) centre (2.4652, -27.6731) ccw
  arc A36 (20.0404, -21.6024) -> (21.6024, -20.0404) centre (0, 0) ccw
  arc A37 (15.3497, -18.9766) -> (20.0404, -21.6024) centre (27.6731, -2.4652) ccw
  arc A38 (14.3572, -19.7382) -> (15.3497, -18.9766) centre (0, 0) ccw
  arc A39 (15.6795, -24.9487) -> (14.3572, -19.7382) centre (-4.7811, -27.3682) ccw
  arc A40 (13.7664, -26.0532) -> (15.6795, -24.9487) centre (0, 0) ccw
  arc A41 (9.9152, -22.3028) -> (13.7664, -26.0532) centre (26.0921, -9.5435) ccw
  arc A42 (8.7594, -22.7816) -> (9.9152, -22.3028) centre (0, 0) ccw
  arc A43 (8.6881, -28.1567) -> (8.7594, -22.7816) centre (-11.7016, -25.1982) ccw
  arc A44 (6.5543, -28.7285) -> (8.6881, -28.1567) centre (0, 0) ccw
  arc A45 (3.805, -24.1091) -> (6.5543, -28.7285) centre (22.733, -15.9715) ccw
  arc A46 (2.5646, -24.2724) -> (3.805, -24.1091) centre (0, 0) ccw
  arc A47 (1.1045, -29.446) -> (2.5646, -24.2724) centre (-17.8247, -21.311) ccw
  arc A48 (-1.1045, -29.446) -> (1.1045, -29.446) centre (0, 0) ccw
  arc A49 (-2.5646, -24.2724) -> (-1.1045, -29.446) centre (17.8247, -21.311) ccw
  arc A50 (-3.805, -24.1091) -> (-2.5646, -24.2724) centre (0, 0) ccw
  arc A51 (-6.5543, -28.7285) -> (-3.805, -24.1091) centre (-22.733, -15.9715) ccw
  arc A52 (-8.6881, -28.1567) -> (-6.5543, -28.7285) centre (0, 0) ccw
  arc A53 (-8.7594, -22.7816) -> (-8.6881, -28.1567) centre (11.7016, -25.1982) ccw
  arc A54 (-9.9152, -22.3028) -> (-8.7594, -22.7816) centre (0, 0) ccw
  arc A55 (-13.7664, -26.0532) -> (-9.9152, -22.3028) centre (-26.0921, -9.5435) ccw
  arc A56 (-15.6795, -24.9487) -> (-13.7664, -26.0532) centre (0, 0) ccw
  arc A57 (-14.3572, -19.7382) -> (-15.6795, -24.9487) centre (4.7811, -27.3682) ccw
  arc A58 (-15.3497, -18.9766) -> (-14.3572, -19.7382) centre (0, 0) ccw
  arc A59 (-20.0404, -21.6024) -> (-15.3497, -18.9766) centre (-27.6731, -2.4652) ccw
  arc A60 (-21.6024, -20.0404) -> (-20.0404, -21.6024) centre (0, 0) ccw
  arc A61 (-18.9766, -15.3497) -> (-21.6024, -20.0404) centre (-2.4652, -27.6731) ccw
  arc A62 (-19.7382, -14.3572) -> (-18.9766, -15.3497) centre (0, 0) ccw
  arc A63 (-24.9487, -15.6795) -> (-19.7382, -14.3572) centre (-27.3682, 4.7811) ccw
  arc A64 (-26.0532, -13.7664) -> (-24.9487, -15.6795) centre (0, 0) ccw
  arc A65 (-22.3028, -9.9152) -> (-26.0532, -13.7664) centre (-9.5435, -26.0921) ccw
  arc A66 (-22.7816, -8.7594) -> (-22.3028, -9.9152) centre (0, 0) ccw
  arc A67 (-28.1567, -8.6881) -> (-22.7816, -8.7594) centre (-25.1982, 11.7016) ccw
  arc A68 (-28.7285, -6.5543) -> (-28.1567, -8.6881) centre (0, 0) ccw
  arc A69 (-24.1091, -3.805) -> (-28.7285, -6.5543) centre (-15.9715, -22.733) ccw
  arc A70 (-24.2724, -2.5646) -> (-24.1091, -3.805) centre (0, 0) ccw
  arc A71 (-29.446, -1.1045) -> (-24.2724, -2.5646) centre (-21.311, 17.8247) ccw
  arc A72 (-29.446, 1.1045) -> (-29.446, -1.1045) centre (0, 0) ccw
  arc A73 (-24.2724, 2.5646) -> (-29.446, 1.1045) centre (-21.311, -17.8247) ccw
  arc A74 (-24.1091, 3.805) -> (-24.2724, 2.5646) centre (0, 0) ccw
  arc A75 (-28.7285, 6.5543) -> (-24.1091, 3.805) centre (-15.9715, 22.733) ccw
  arc A76 (-28.1567, 8.6881) -> (-28.7285, 6.5543) centre (0, 0) ccw
  arc A77 (-22.7816, 8.7594) -> (-28.1567, 8.6881) centre (-25.1982, -11.7016) ccw
  arc A78 (-22.3028, 9.9152) -> (-22.7816, 8.7594) centre (0, 0) ccw
  arc A79 (-26.0532, 13.7664) -> (-22.3028, 9.9152) centre (-9.5435, 26.0921) ccw
  arc A80 (-24.9487, 15.6795) -> (-26.0532, 13.7664) centre (0, 0) ccw
  arc A81 (-19.7382, 14.3572) -> (-24.9487, 15.6795) centre (-27.3682, -4.7811) ccw
  arc A82 (-18.9766, 15.3497) -> (-19.7382, 14.3572) centre (0, 0) ccw
  arc A83 (-21.6024, 20.0404) -> (-18.9766, 15.3497) centre (-2.4652, 27.6731) ccw
  arc A84 (-20.0404, 21.6024) -> (-21.6024, 20.0404) centre (0, 0) ccw
  arc A85 (-15.3497, 18.9766) -> (-20.0404, 21.6024) centre (-27.6731, 2.4652) ccw
  arc A86 (-14.3572, 19.7382) -> (-15.3497, 18.9766) centre (0, 0) ccw
  arc A87 (-15.6795, 24.9487) -> (-14.3572, 19.7382) centre (4.7811, 27.3682) ccw
  arc A88 (-13.7664, 26.0532) -> (-15.6795, 24.9487) centre (0, 0) ccw
  arc A89 (-9.9152, 22.3028) -> (-13.7664, 26.0532) centre (-26.0921, 9.5435) ccw
  arc A90 (-8.7594, 22.7816) -> (-9.9152, 22.3028) centre (0, 0) ccw
  arc A91 (-8.6881, 28.1567) -> (-8.7594, 22.7816) centre (11.7016, 25.1982) ccw
  arc A92 (-6.5543, 28.7285) -> (-8.6881, 28.1567) centre (0, 0) ccw
  arc A93 (-3.805, 24.1091) -> (-6.5543, 28.7285) centre (-22.733, 15.9715) ccw
  arc A94 (-2.5646, 24.2724) -> (-3.805, 24.1091) centre (0, 0) ccw
  arc A95 (-1.1045, 29.446) -> (-2.5646, 24.2724) centre (17.8247, 21.311) ccw
  circle A96 centre (0, 0) radius 5.22
  circle A97 centre (-12, 12) radius 2.72
  circle A98 centre (-12, -12) radius 2.72
  circle A99 centre (12, 12) radius 2.72
  circle A100 centre (12, -12) radius 2.72
equation "\"d0\" = da_da"
equation "\"d1\" = da_b"
equation "\"d3\" = da_dw"
equation "\"da_da\" = 58.493319"
equation "\"da_b\" = 20"
equation "\"da_dw\" = 54.193548"
body "Solid1"
body "Srf1"
